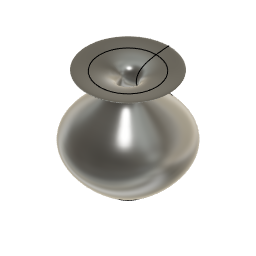
vase (Autodesk Fusion 360 design; units mm, degrees)
Autodesk Fusion 360 part; units mm, degrees
sketch "vase_side_sketch" plane through (0, 0, 0) normal (1, 0, 0) x (0, 1, 0)
  spline S0 degree 5 poles (22.9536, 74.4897) (20.9764, 74.2046) (17.4742, 73.559) (13.578, 72.3642) (10.98, 70.3368) (11.375, 67.175) (14.502, 63.497) (19.398, 59.3889) (25.1275, 54.9037) (30.8101, 50.0718) (35.6639, 44.9073) (39.0399, 39.4155) (40.4756, 33.6025) (39.723, 27.4815) (36.6755, 21.0675) (31.3206, 14.3755) (25.2188, 8.8091) (19.6406, 4.5182) (15.4796, 1.6064) (13.2887, 0.1377) knots 0 0 0 0 0 0 0.066667 0.133333 0.2 0.266667 0.333333 0.4 0.466667 0.533333 0.6 0.666667 0.733333 0.8 0.866667 0.933333 1 1 1 1 1 1
  line L0 (45.5983, 77.7548) -> (0.309, 71.2247)
  spline S1 degree 3 poles (22.2401, 79.4386) (18.935, 78.962) (16.2245, 78.3685) (13.9166, 77.5124) (12.3313, 76.9244) (10.9102, 76.2187) (9.6293, 75.1464) (8.6764, 74.3487) (7.7985, 73.306) (7.2345, 72.0346) (6.6843, 70.7943) (6.4881, 69.3809) (6.6043, 68.1331) (6.7466, 66.6053) (7.2705, 65.3354) (7.8827, 64.2484) (8.827, 62.5716) (10.0221, 61.2326) (11.3503, 59.9117) (13.6175, 57.6571) (16.3341, 55.5015) (19.1092, 53.2606) (22.8137, 50.2693) (26.5832, 47.1594) (29.4007, 44.0767) (31.4949, 41.7854) (33.0446, 39.5341) (33.9372, 37.4217) (34.8417, 35.281) (35.1402, 33.2999) (34.8538, 31.0942) (34.5693, 28.9027) (33.6528, 26.4276) (31.8406, 23.6202) (29.1405, 19.4371) (24.4476, 14.619) (17.7819, 9.4963) (15.5695, 7.796) (13.1427, 6.0593) (10.5046, 4.2909) knots 0 0 0 0 0.0625 0.0625 0.0625 0.105429 0.105429 0.105429 0.137366 0.137366 0.137366 0.168521 0.168521 0.168521 0.206666 0.206666 0.206666 0.265502 0.265502 0.265502 0.365927 0.365927 0.365927 0.499979 0.499979 0.499979 0.599616 0.599616 0.599616 0.700589 0.700589 0.700589 0.80091 0.80091 0.80091 0.950386 0.950386 0.950386 1 1 1 1
  spline S2 degree 5 poles (22.2401, 79.4386) (23.7381, 79.6436) (26.4626, 79.9997) (29.734, 80.3716) (32.4446, 80.5388) (33.0191, 80.1871) (31.0247, 79.3206) (27.017, 78.0456) (22.7341, 76.6979) (19.7217, 75.5774) (18.5456, 74.7953) (19.278, 74.4808) (20.7583, 74.4186) (22.1538, 74.4533) (22.9536, 74.4897) knots 0 0 0 0 0 0 0.1 0.2 0.3 0.4 0.5 0.6 0.7 0.8 0.9 1 1 1 1 1 1
  line L1 (29.6027, 78.88) -> (24.98, 77.3954)
  line L2 (13.2887, 0.1377) -> (0.009, 0.1377)
  line L3 (10.5046, 4.2909) -> (0.009, 4.2909)
  line L4 (0.009, 4.2909) -> (0.009, 0.1377)
  point P0 (12.8541, 65.7548)
  point P1 (37.9703, 40.607)
  point P2 (27.2913, 78.1377)
  dimension "d1" = 5
  constraint midpoint S0.start L0
  constraint midpoint P2 L1
  constraint horizontal L2
  constraint horizontal L3
  constraint perpendicular L2 L4
revolve "Revolve1" add sketch "vase_side_sketch" angle 360 about axis through (0, 0, 1.75) along (0, 0, 1)
delete_face "DeleteFace1" 1 faces at (-0.0051, 0.0075, 2.9065)
named bodies: "vase"
